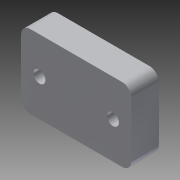
# Autodesk Inventor part: Spacer 3
Saved by Autodesk Inventor 2014 SP1 (Build 180222100, 222)
## iProperties
Created: 2014-01-14
Part Number: Spacer 3
Material: Aluminum 6061
Document SubType Name: Modeling
Designer: Arpan
Density: 2.71 g/cm^3
Appearance: Aluminum - Flat
Author: Arpan
Autodesk Inventor part; units mm, degrees
ref_plane "YZ Plane" through (0, 0, 0) normal (1, 0, 0) x (0, 1, 0)
ref_plane "XZ Plane" through (0, 0, 0) normal (0, 1, 0) x (-1, 0, 0)
ref_plane "XY Plane" through (0, 0, 0) normal (0, 0, 1) x (1, 0, 0)
sketch "Sketch1" plane through (0, 0, 0) normal (0, 0, 1) x (1, 0, 0)
  line L0 (3.175, 0) -> (34.925, 0)
  line L1 (38.1, 3.175) -> (38.1, 22.225)
  line L2 (34.925, 25.4) -> (3.175, 25.4)
  line L3 (0, 22.225) -> (0, 3.175)
  circle A0 centre (6.35, 12.7) radius 2.0701
  circle A1 centre (31.75, 12.7) radius 2.0701
  arc A2 (3.175, 25.4) -> (0, 22.225) centre (3.175, 22.225) ccw
  arc A3 (38.1, 22.225) -> (34.925, 25.4) centre (34.925, 22.225) ccw
  arc A4 (34.925, 0) -> (38.1, 3.175) centre (34.925, 3.175) ccw
  arc A5 (0, 3.175) -> (3.175, 0) centre (3.175, 3.175) ccw
  point P0 (0, 0)
  point P1 (38.1, 25.4)
  point P2 (38.1, 0)
  point P3 (0, 25.4)
  dimension "d0" = 38.1
  dimension "d1" = 25.4
  dimension "d2" = 4.1402
  dimension "d3" = 12.7
  dimension "d4" = 6.35
  dimension "d7" = 25.4
  dimension "d21" = 3.175
  constraints: 8 end point, 8 point on circle, 8 point on line, 8 tangent, 6 centre point, 3 equal radius, 2 horizontal, 2 parallel, 1 perpendicular, 2 other
  measures "d0" distance of point (0, 25.4) point (38.1, 25.4)
  measures "d1" distance of point (38.1, 25.4) point (38.1, 0)
  measures "d2" diameter of A0
  measures "d3" distance from line of L0 A0.centre
  measures "d4" distance from line of L3 A0.centre
  measures "d7" distance of A0.centre A1.centre
  measures "d21" radius of A2
extrude "Extrusion1" add sketch "Sketch1" along normal blind 9.525
body "Solid1"
